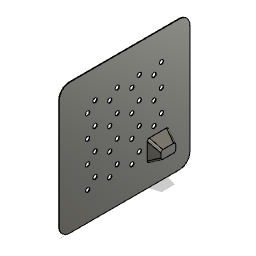
pyramid grid v2 (Autodesk Fusion 360 design; units mm, degrees)
Autodesk Fusion 360 part; units mm, degrees
sketch "peg" plane through (0, 0, 0) normal (1, 0, 0) x (0, 0, -1)
  line L0 (10, 10) -> (-10, 10)
  line L1 (-10, 10) -> (-10, -10)
  line L2 (-10, -10) -> (10, -10)
  line L3 (10, -10) -> (10, 10)
  line L4 (10, 10) -> (-10, -10) construction
  line L5 (-10, 10) -> (10, -10) construction
  circle A0 centre (3.5355, 3.5355) radius 2
  circle A1 centre (-3.5355, -3.5355) radius 2
  line L6 (7.5, 7.5) -> (-7.5, 7.5)
  line L7 (-7.5, 7.5) -> (-7.5, -7.5)
  line L8 (-7.5, -7.5) -> (7.5, -7.5)
  line L9 (7.5, -7.5) -> (7.5, 7.5)
  line L10 (7.5, 7.5) -> (-7.5, -7.5) construction
  line L11 (-7.5, 7.5) -> (7.5, -7.5) construction
  line L12 (10.5, -10.5) -> (-10.5, -10.5)
  line L13 (-10.5, -10.5) -> (-10.5, 10.5)
  line L14 (-10.5, 10.5) -> (10.5, 10.5)
  line L15 (10.5, 10.5) -> (10.5, -10.5)
  line L16 (10.5, -10.5) -> (-10.5, 10.5) construction
  line L17 (-10.5, -10.5) -> (10.5, 10.5) construction
  dimension "d1" = 20
  dimension "d2" = 20
  dimension "d3" = 4
  dimension "d4" = 4
  dimension "d5" = 5
  dimension "d6" = 5
  dimension "d7" = 15
  dimension "d8" = 15
  dimension "d23" = 21
  dimension "d24" = 21
  constraint horizontal L0
  constraint perpendicular L0 L1
  constraint parallel L0 L2
  constraint parallel L1 L3
  constraint coincident L4 origin
  constraint coincident L5 origin
  constraint coincident L4 A0.centre
  constraint coincident L4 A1.centre
  constraint horizontal L6
  constraint perpendicular L6 L7
  constraint parallel L6 L8
  constraint parallel L7 L9
  constraint coincident L10 origin
  constraint coincident L11 origin
  constraint horizontal L12
  constraint perpendicular L12 L13
  constraint parallel L12 L14
  constraint parallel L13 L15
  constraint coincident L16 origin
  constraint coincident L17 origin
  measures "d1" distance of L1.end L2.end
  measures "d2" distance of L0.end L1.end
  measures "d3" diameter of A0
  measures "d4" diameter of A1
  measures "d5" distance of origin A0.centre
  measures "d6" distance of origin A1.centre
  measures "d7" distance of L7.end L8.end
  measures "d8" distance of L6.end L7.end
  measures "d23" distance of L13.end L14.end
  measures "d24" distance of L12.end L13.end
extrude "Extrude1" add sketch "peg" along normal blind 10 contours L0 L1 L2 L3 | A0 | A1 | L6 L7 L8 L9 makes body 1
extrude "Extrude2" add sketch "peg" against normal blind 3.5 contours A0 | A1 bodies 1
extrude "Extrude3" add sketch "peg" against normal blind 2 from surface at -0.5 separate body contours L6 L7 L8 L9 makes body 2
move_face "OffsetFaces1" offset -0.1 2 faces at (-1.8333, 3.4358, -5.533) (-1.8333, -3.6352, 1.538) on bodies 2
chamfer "Chamfer1" distance 1 angle 45 2 edges at (-2.5, 2.7761, -1.5776) (-2.5, -4.2949, 5.4934) on bodies 2
chamfer "Chamfer2" distance 3 distance2 10 2 edges at (10, 0, -10) (10, 0, 10) measured on face at (10, 3.3333, 3.3333) measured on face at (10, 3.3333, 3.3333) on bodies 1
chamfer "Chamfer3" distance 6 distance2 10 2 edges at (10, 10, 0) (10, -10, 0) measured on face at (10, -3.3333, 2.3335) measured on face at (10, -3.3333, 2.3335) on bodies 1
fillet "Fillet1" radius 2 4 edges at (5, 7, -8.5) (5, -7, -8.5) (5, -7, 8.5) (5, 7, 8.5) on bodies 1
extrude "Extrude4" add sketch "peg" against normal blind 0.5 separate body contours L0 L1 L2 L3 | L6 L7 L8 L9 | L12 L13 L14 L15 makes body 3
pattern_linear "R-Pattern1" count 4 spacing 21 along (0, 1, 0) count 4 spacing 21 along (0, 0, 1) of bodies 3 makes body 4 at (0, 16.7507, -4.3076) makes body 5 at (0, 37.7507, -4.3076) makes body 6 at (0, 67.2493, 4.3076) makes body 7 at (0, -4.2493, 16.6924) makes body 8 at (0, 16.7507, 16.6924) makes body 9 at (0, 37.7507, 16.6924) makes body 10 at (0, 58.7507, 16.6924) makes body 11 at (0, -4.2493, 37.6924) makes body 12 at (0, 16.7507, 37.6924) makes body 13 at (0, 37.7507, 37.6924) makes body 14 at (0, 67.2493, 46.3076) makes body 15 at (0, -4.2493, 58.6924) makes body 16 at (0, 16.7507, 58.6924) makes body 17 at (0, 37.7507, 58.6924) makes body 18 at (0, 58.7507, 58.6924)
combine "Combine1" operation add target body 3 tool bodies 4 6 15 17 16 9 7 8 10 11 12 13 5 14 18
sketch "fabric outline" plane through (0, 0, 0) normal (1, 0, 0) x (0, 0, -1)
  circle A0 centre (-59.4645, 66.5355) radius 2
  circle A1 centre (-66.5355, 59.4645) radius 2
  circle A2 centre (-38.4645, 66.5355) radius 2
  circle A3 centre (-45.5355, 59.4645) radius 2
  circle A4 centre (3.5355, 45.5355) radius 2
  circle A5 centre (-3.5355, 38.4645) radius 2
  circle A6 centre (-38.4645, 45.5355) radius 2
  circle A7 centre (-45.5355, 38.4645) radius 2
  circle A8 centre (-38.4645, 24.5355) radius 2
  circle A9 centre (-45.5355, 17.4645) radius 2
  circle A10 centre (-59.4645, 3.5355) radius 2
  circle A11 centre (-66.5355, -3.5355) radius 2
  circle A12 centre (-59.4645, 24.5355) radius 2
  circle A13 centre (-66.5355, 17.4645) radius 2
  circle A14 centre (-66.5355, 38.4645) radius 2
  circle A15 centre (-59.4645, 45.5355) radius 2
  circle A16 centre (-45.5355, -3.5355) radius 2
  circle A17 centre (-38.4645, 3.5355) radius 2
  circle A18 centre (3.5355, 66.5355) radius 2
  circle A19 centre (-3.5355, 59.4645) radius 2
  circle A20 centre (-24.5355, 59.4645) radius 2
  circle A21 centre (-17.4645, 66.5355) radius 2
  circle A22 centre (-17.4645, 45.5355) radius 2
  circle A23 centre (-24.5355, 38.4645) radius 2
  circle A24 centre (-24.5355, 17.4645) radius 2
  circle A25 centre (-17.4645, 24.5355) radius 2
  circle A26 centre (-17.4645, 3.5355) radius 2
  circle A27 centre (-24.5355, -3.5355) radius 2
  circle A28 centre (3.5355, 24.5355) radius 2
  circle A29 centre (-3.5355, 17.4645) radius 2
  circle A30 centre (-3.5355, -3.5355) radius 2
  circle A31 centre (3.5355, 3.5355) radius 2
  line L0 (-73.5, -10.5) -> (10.5, -10.5)
  line L1 (10.5, -10.5) -> (10.5, 73.5)
  line L2 (10.5, 73.5) -> (-73.5, 73.5)
  line L3 (-73.5, 73.5) -> (-73.5, -10.5)
  circle A32 centre (-59.4645, 66.5355) radius 2
  circle A33 centre (-66.5355, 59.4645) radius 2
  circle A34 centre (-38.4645, 66.5355) radius 2
  circle A35 centre (-45.5355, 59.4645) radius 2
  circle A36 centre (3.5355, 45.5355) radius 2
  circle A37 centre (-3.5355, 38.4645) radius 2
  circle A38 centre (-38.4645, 45.5355) radius 2
  circle A39 centre (-45.5355, 38.4645) radius 2
  circle A40 centre (-38.4645, 24.5355) radius 2
  circle A41 centre (-45.5355, 17.4645) radius 2
  circle A42 centre (-38.4645, 3.5355) radius 2
  circle A43 centre (-45.5355, -3.5355) radius 2
  circle A44 centre (-59.4645, 24.5355) radius 2
  circle A45 centre (-66.5355, 17.4645) radius 2
  circle A46 centre (-59.4645, 45.5355) radius 2
  circle A47 centre (-66.5355, 38.4645) radius 2
  circle A48 centre (-59.4645, 3.5355) radius 2
  circle A49 centre (-66.5355, -3.5355) radius 2
  line L4 (-73.5, -10.5) -> (-73.5, 73.5)
  circle A50 centre (-17.4645, 66.5355) radius 2
  circle A51 centre (-24.5355, 59.4645) radius 2
  circle A52 centre (-17.4645, 24.5355) radius 2
  circle A53 centre (-24.5355, 17.4645) radius 2
  circle A54 centre (-17.4645, 3.5355) radius 2
  circle A55 centre (-24.5355, -3.5355) radius 2
  circle A56 centre (-17.4645, 45.5355) radius 2
  circle A57 centre (-24.5355, 38.4645) radius 2
  circle A58 centre (3.5355, 24.5355) radius 2
  circle A59 centre (-3.5355, 17.4645) radius 2
  circle A60 centre (3.5355, 3.5355) radius 2
  circle A61 centre (-3.5355, -3.5355) radius 2
  line L5 (10.5, -10.5) -> (-73.5, -10.5)
  line L6 (10.5, 73.5) -> (10.5, -10.5)
  circle A62 centre (3.5355, 66.5355) radius 2
  circle A63 centre (-3.5355, 59.4645) radius 2
  line L7 (-73.5, 73.5) -> (10.5, 73.5)
  line L8 (30.5, -30.5) -> (-93.5, -30.5)
  line L9 (-93.5, -30.5) -> (-93.5, 93.5)
  line L10 (-93.5, 93.5) -> (30.5, 93.5)
  line L11 (30.5, 93.5) -> (30.5, -30.5)
  dimension "d32" = -20
extrude "Extrude5" add sketch "fabric outline" against normal blind 0.5 contours L8 L9 L10 L11 bodies 3
fillet "Fillet2" radius 10 4 edges at (-0.25, 93.5, -30.5) (-0.25, 93.5, 93.5) (-0.25, -30.5, -30.5) (-0.25, -30.5, 93.5) on bodies 3
sketch "pyramid grid fabric" plane through (0, 0, 0) normal (1, 0, 0) x (0, 0, -1)
  arc A0 (-93.5, -20.5) -> (-83.5, -30.5) centre (-83.5, -20.5) ccw
  line L0 (20.5, -30.5) -> (-83.5, -30.5)
  arc A1 (20.5, -30.5) -> (30.5, -20.5) centre (20.5, -20.5) ccw
  arc A2 (-83.5, 93.5) -> (-93.5, 83.5) centre (-83.5, 83.5) ccw
  line L1 (-83.5, 93.5) -> (20.5, 93.5)
  arc A3 (30.5, 83.5) -> (20.5, 93.5) centre (20.5, 83.5) ccw
  line L2 (-93.5, -20.5) -> (-93.5, 83.5)
  line L3 (30.5, 83.5) -> (30.5, -20.5)
  circle A4 centre (-59.4645, 66.5355) radius 2
  circle A5 centre (-66.5355, 59.4645) radius 2
  circle A6 centre (-38.4645, 66.5355) radius 2
  circle A7 centre (-45.5355, 59.4645) radius 2
  circle A8 centre (3.5355, 45.5355) radius 2
  circle A9 centre (-3.5355, 38.4645) radius 2
  circle A10 centre (-38.4645, 45.5355) radius 2
  circle A11 centre (-45.5355, 38.4645) radius 2
  circle A12 centre (-38.4645, 24.5355) radius 2
  circle A13 centre (-45.5355, 17.4645) radius 2
  circle A14 centre (-38.4645, 3.5355) radius 2
  circle A15 centre (-45.5355, -3.5355) radius 2
  circle A16 centre (-59.4645, 24.5355) radius 2
  circle A17 centre (-66.5355, 17.4645) radius 2
  circle A18 centre (-59.4645, 45.5355) radius 2
  circle A19 centre (-66.5355, 38.4645) radius 2
  circle A20 centre (-59.4645, 3.5355) radius 2
  circle A21 centre (-66.5355, -3.5355) radius 2
  circle A22 centre (-17.4645, 66.5355) radius 2
  circle A23 centre (-24.5355, 59.4645) radius 2
  circle A24 centre (-17.4645, 24.5355) radius 2
  circle A25 centre (-24.5355, 17.4645) radius 2
  circle A26 centre (-17.4645, 3.5355) radius 2
  circle A27 centre (-24.5355, -3.5355) radius 2
  circle A28 centre (-17.4645, 45.5355) radius 2
  circle A29 centre (-24.5355, 38.4645) radius 2
  circle A30 centre (3.5355, 24.5355) radius 2
  circle A31 centre (-3.5355, 17.4645) radius 2
  circle A32 centre (3.5355, 3.5355) radius 2
  circle A33 centre (-3.5355, -3.5355) radius 2
  circle A34 centre (3.5355, 66.5355) radius 2
  circle A35 centre (-3.5355, 59.4645) radius 2
fillet "Fillet3" radius 3 4 edges at (-1.5, 7.5, -7.5) (-1.5, 7.5, 7.5) (-1.5, -7.5, -7.5) (-1.5, -7.5, 7.5) on bodies 2
named bodies: "pyramid grid pyramid", "pyramid grid back", "fabric", "fabric (1)", "fabric (2)", "fabric (3)", "fabric (4)", "fabric (5)", "fabric (6)", "fabric (7)", "fabric (8)", "fabric (9)", "fabric (10)", "fabric (11)", "fabric (12)", "fabric (13)", "fabric (14)", "fabric (15)"
